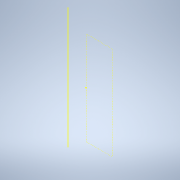
# Autodesk Inventor part: Part1
Saved by Autodesk Inventor 2021 (Build 250183000, 183)
## iProperties
Created: 2021-01-21
Part Number: Part1
Material: Generic
Document SubType Name: Modeling
Designer: Sam
Density: 1 g/cm^3
Appearance: Default
Author: Sam
Autodesk Inventor part; units mm, degrees
ref_plane "YZ Plane" through (0, 0, 0) normal (1, 0, 0) x (0, 1, 0)
sketch "Sketch3" plane through (0, 0, 0) normal (0, 0, 1) x (1, 0, 0)
  line L0 (-5, 9) -> (-5, -9) construction
  line L1 (0, -9) -> (0, 9) construction
  line L2 (0, -9) -> (-5, -9) construction
  line L3 (0, 9) -> (-5, 9) construction
  line L4 (22.41, -1.9333) -> (22.41, 7.875) construction
  line L5 (0, 0) -> (32.457, 0)
  line L6 (-5, 9) -> (0, 9)
  line L7 (0, 8) -> (0, 9)
  line L8 (0, 8) -> (17.41, 8)
  line L9 (17.41, 8) -> (17.41, 0)
  line L10 (22.41, 0) -> (22.41, 12)
  line L11 (22.41, 12) -> (-8, 12)
  line L12 (-8, 12) -> (-8, 9)
  line L13 (-8, 9) -> (-5, 9)
  line L14 (0, -9) -> (-5, -9) construction
  line L15 (-5, -9) -> (0, -9)
  line L16 (0, -8) -> (0, -9)
  line L17 (0, -8) -> (17.41, -8)
  line L18 (17.41, -8) -> (17.41, 0)
  line L19 (22.41, 0) -> (22.41, -12)
  line L20 (22.41, -12) -> (-8, -12)
  line L21 (-8, -12) -> (-8, -9)
  line L22 (-8, -9) -> (-5, -9)
  point P0 (22.41, -7.875)
  dimension "d11" = 3
  dimension "d12" = 3
  dimension "d13" = 4
  dimension "d14" = 5
  constraints: 36 end point, 6 symmetric about line, 5 point on line, 3 perpendicular, 2 collinear, 2 horizontal, 1 vertical
  measures "d11" distance between parallel lines of L11 L13
  measures "d12" distance between parallel lines of L0 L12
  measures "d13" distance between parallel lines of L11 L8
  measures "d14" distance from line of L4.end L9
extrude "Extrusion3" add sketch "Sketch3" along normal mid plane 10
sketch "Sketch4" plane through (22.41, -12, 5) normal (1, 0, 0) x (0, 0, -1)
  line L0 (5, 12) -> (5, -10.2274)
  line L1 (10, 3) -> (-5, 3)
  line L2 (-5, 3) -> (-5, 12)
  line L3 (0, 21) -> (15, 21)
  line L4 (15, 21) -> (15, 12)
  line L5 (10, 0) -> (0, 0) projected
  line L6 (10, 24) -> (0, 24) projected
  line L7 (10, 3) -> (0, 3) projected
  line L8 (10, 3) -> (10, 12)
  line L9 (10, 4) -> (10, 20) projected
  line L10 (15, 12) -> (10, 12)
  line L11 (0, 24) -> (0, 21) projected
  line L12 (0, 21) -> (0, 12)
  line L13 (0, 20) -> (0, 4) projected
  line L14 (-5, 12) -> (0, 12)
  dimension "d17" = 20
  dimension "d18" = 3
  dimension "d19" = 3
  dimension "d40" = 9
  dimension "d41" = 9
  constraints: 18 end point, 5 perpendicular, 2 midpoint, 2 point on line, 1 horizontal, 1 vertical, 1 other
  measures "d17" distance between parallel lines of L2 L4
  measures "d18" distance between parallel lines of L1 L5
  measures "d19" distance between parallel lines of L6 L3
  measures "d40" distance between parallel lines of L1 L14
  measures "d41" distance between parallel lines of L3 L10
extrude "Extrusion4" add sketch "Sketch4" against normal up to surface (5 mm away)
sketch "Sketch5" plane through (17.41, -8, -5) normal (-1, 0, 0) x (0, 0, 1)
  circle A0 centre (-1.0339, 12.225) radius 1.15 projected
  circle A1 centre (11.0339, 3.775) radius 1.15 projected
  point P0 (5, 8)
  constraints: 2 coincident
hole "Hole1" at (17.41, 4.225, -6.0339) at (17.41, -4.225, 6.0339) direction (1, 0, 0) diameter 3 end through all
sketch "Sketch6" plane through (17.41, -8, -5) normal (-1, 0, 0) x (0, 0, 1)
  circle A0 centre (-1.0339, 12.225) radius 1.5 projected
  circle A1 centre (11.0339, 3.775) radius 1.5 projected
  line L0 (1.8529, 12.225) -> (0.4095, 9.725)
  line L1 (0.4095, 9.725) -> (-2.4772, 9.725)
  line L2 (-2.4772, 9.725) -> (-3.9206, 12.225)
  line L3 (-3.9206, 12.225) -> (-2.4772, 14.725)
  line L4 (-2.4772, 14.725) -> (0.4095, 14.725)
  line L5 (0.4095, 14.725) -> (1.8529, 12.225)
  line L6 (13.9206, 3.775) -> (12.4772, 1.275)
  line L7 (12.4772, 1.275) -> (9.5905, 1.275)
  line L8 (9.5905, 1.275) -> (8.1471, 3.775)
  line L9 (8.1471, 3.775) -> (9.5905, 6.275)
  line L10 (9.5905, 6.275) -> (12.4772, 6.275)
  line L11 (12.4772, 6.275) -> (13.9206, 3.775)
  point P0 (5, 8)
  dimension "d29" = 5
  constraints: 24 end point, 2 coincident, 2 horizontal alignment, 1 parallel, 26 other
  measures "d29" distance between parallel lines of L7 L10
extrude "Extrusion5" cut sketch "Sketch6" against normal blind 3.5
ref_plane "Work Plane1" through (17.41, 2.975, -3.8688) normal (0, -0.8660254, -0.5) x (1, 0, 0)
ref_plane "Work Plane2" through (0, -9, 21.3253) normal (0, -1, 0) x (0, 0, 1)
sketch "Sketch7" plane through (0, -10.9282, 20.2121) normal (0, -0.8660254, -0.5) x (0, -0.5, 0.8660254)
  line L0 (-32.8062, -17.41) -> (-32.8062, -20.91) projected
  line L1 (-32.8062, -17.41) -> (-32.8062, -20.91) projected
  line L2 (-27.8062, -17.41) -> (-27.8062, -20.91) projected
  line L3 (-27.8062, -17.41) -> (-27.8062, -20.91) projected
  line L4 (-28.8062, -20.91) -> (-31.8062, -20.91) projected
  line L5 (-30.3062, -20.91) -> (-30.3062, -15.0527)
  line L6 (-32.8062, -17.41) -> (-32.8062, -20.91) projected
  line L7 (-32.8062, -17.41) -> (-30.3062, -17.41) projected
  arc A0 (-32.8062, -18.61) -> (-32.8062, -17.41) centre (-33.6062, -18.01) ccw
  line L8 (-32.8062, -17.41) -> (-32.8062, -18.61)
  arc A1 (-27.8062, -17.41) -> (-27.8062, -18.61) centre (-27.0062, -18.01) ccw
  line L9 (-27.8062, -17.41) -> (-27.8062, -18.61)
  point P0 (-22.9683, 0)
  point P1 (-32.6062, -18.01)
  point P2 (-28.0062, -18.01)
  dimension "d32" = 0.2
  dimension "d33" = 1.2
  constraints: 6 end point, 5 point on circle, 5 symmetric about line, 2 centre point, 1 collinear, 1 horizontal alignment, 1 midpoint, 1 point on line, 1 vertical, 1 other
  measures "d32" distance from line of L0 point (-32.606, -18.01)
  measures "d33" distance of L8.end L1.start
sketch "Sketch8" plane through (0, 0, 0) normal (0, 0, -1) x (-1, 0, 0)
  line L0 (0, 9) -> (7.2, 9) projected
  arc A0 (5.2, 9) -> (7.2, 9) centre (6.2, 10.05) ccw
  line L1 (5, -9) -> (5, 9) projected
  line L2 (7.2, 9) -> (0, 9) projected
  line L3 (7.2, 9) -> (5.2, 9)
  line L4 (0, 0) -> (12.0041, 0)
  arc A1 (7.2, -9) -> (5.2, -9) centre (6.2, -10.05) ccw
  line L5 (7.2, -9) -> (5.2, -9)
  line L6 (8, 9) -> (8, 12) projected
  point P0 (6.2, 8.6)
  point P1 (6.2, -8.6)
  dimension "d34" = 0.4
  dimension "d35" = 2
  dimension "d36" = 0.8
  constraints: 6 end point, 5 point on circle, 4 symmetric about line, 2 centre point, 2 horizontal, 1 point on line, 1 vertical alignment, 1 other
  measures "d34" distance from line of L0 point (6.2, 8.6)
  measures "d35" distance of L3.end L0.end
  measures "d36" distance from line of L6 L0.end
extrude "Extrusion6" add sketch "Sketch8" along normal mid plane 6
fillet "Fillet1" radius 0.7 2 edges at (-8, 9, 0) (-8, -9, 0)
fillet "Fillet2" radius 5 2 edges at (19.91, 0, -5) (19.91, 0, 5)
fillet "Fillet3" radius 4 2 edges at (19.91, -9, 10) (19.91, 9, -10)
fillet "Fillet4" radius 3 2 edges at (19.91, 9, -5) (19.91, -9, 5)
fillet "Fillet5" radius 2 2 edges at (17.41, 8, 0) (17.41, -8, 0)
body "Solid3"
